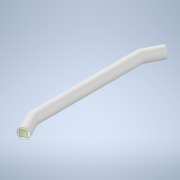
# Autodesk Inventor part: caña bici ruta
Saved by Autodesk Inventor 2021 (Build 250183000, 183)
## iProperties
Created: 2021-07-10
Part Number: caña bici ruta
Material: Generic
Document SubType Name: Modeling
Designer: j2seb
Density: 1 g/cm^3
Appearance: Default
Author: j2seb
Autodesk Inventor part; units mm, degrees
ref_plane "YZ Plane" through (0, 0, 0) normal (1, 0, 0) x (0, 1, 0)
sketch "Sketch1" plane through (0, 0, 0) normal (0, 1, 0) x (-1, 0, 0)
  line L0 (-84.2229, 348.4458) -> (-4.2229, 188.4458)
  line L1 (0, 170.5573) -> (0, 0)
  line L2 (53.8545, 0) -> (-53.8545, 0)
  line L3 (-84.2229, -348.4458) -> (-4.2229, -188.4458)
  line L4 (0, -170.5573) -> (0, 0)
  arc A0 (0, 170.5573) -> (-4.2229, 188.4458) centre (-40, 170.5573) ccw
  arc A1 (-4.2229, -188.4458) -> (0, -170.5573) centre (-40, -170.5573) ccw
  point P0 (0, 180)
  point P1 (0, -180)
  dimension "d0" = 180
  dimension "d1" = 40
  dimension "d2" = 80
  dimension "d3" = 160
  dimension "d8" = 40
  constraints: 10 end point, 4 point on circle, 4 point on line, 4 tangent, 2 centre point, 2 symmetric about line, 1 horizontal, 1 midpoint, 1 vertical
  measures "d0" distance of point (0, 180) L1.end
  measures "d1" radius of A0
  measures "d2" horizontal distance of L0.end L0.start
  measures "d3" vertical distance of L0.start L0.end
  measures "d8" radius of A1
ref_plane "Work Plane1" through (84.2229, 0, 348.4458) normal (-0.4472136, 0, -0.8944272) x (0, -1, 0)
sketch "Sketch2" plane through (84.2229, 0, 348.4458) normal (-0.4472136, 0, -0.8944272) x (0, -1, 0)
  circle A0 centre (0, 0) radius 20
  circle A1 centre (0, 0) radius 18.5
  point P0 (0, -80.4984)
  dimension "d4" = 40
  dimension "d5" = 37
  constraints: 2 centre point, 1 coincident
  measures "d4" diameter of A0
  measures "d5" diameter of A1
sweep "Sweep1" add profiles "Sketch2" path "Sketch1" path curves L0 A0 L1 L4 A1 L3
equation "\"d8\" = d1"
body "Solid1"
